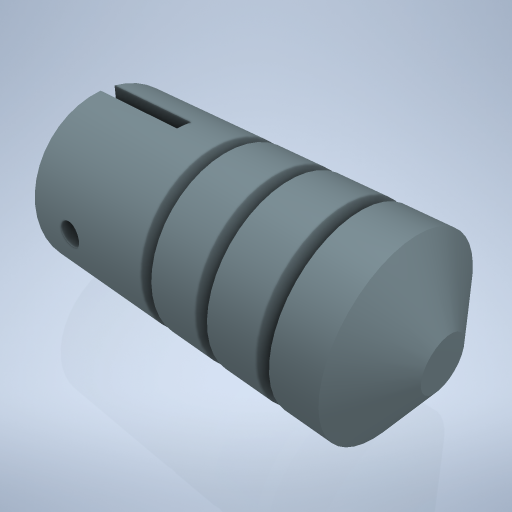
# Autodesk Inventor part: arbeitskolben
Saved by Autodesk Inventor 2024.2 (Build 282272000, 272)
## iProperties
Created: 2024-04-15
Part Number: arbeitskolben
Material: Blei
Document SubType Name: Modeling
Designer: Fabri
Density: 11.34 g/cm^3
Appearance: Blei
Author: Fabri
Autodesk Inventor part; units mm, degrees
ref_plane "YZ Plane" through (0, 0, 0) normal (1, 0, 0) x (0, 1, 0)
ref_plane "XY Plane" through (0, 0, 0) normal (0, 0, 1) x (1, 0, 0)
sketch "Skizze4" plane through (0, 0, 0) normal (0, 0, 1) x (1, 0, 0)
  line L0 (0, 0) -> (0, 7)
  line L1 (0, 7) -> (11.5, 7)
  line L2 (11.5, 7) -> (12, 6.134)
  line L3 (12, 6.134) -> (12.5, 7)
  line L4 (12.5, 7) -> (16.5, 7)
  line L5 (16.5, 7) -> (17, 6.134)
  line L6 (17, 6.134) -> (17.5, 7)
  line L7 (17.5, 7) -> (21.5, 7)
  line L8 (21.5, 7) -> (22, 6.134)
  line L9 (22, 6.134) -> (22.5, 7)
  line L10 (22.5, 7) -> (26.1132, 7)
  line L11 (26.1132, 7) -> (29, 2)
  line L12 (29, 2) -> (29, 0)
  line L13 (29, 0) -> (0, 0)
  line L14 (12, 6.134) -> (12, 7.9514) construction
  line L15 (17, 6.134) -> (17, 8.1262) construction
  line L16 (22, 6.134) -> (22, 7.8166) construction
  point P0 (29, 1)
  dimension "d7" = 1
  dimension "d8" = 60
  dimension "d9" = 4
  dimension "d10" = 14
  dimension "d11" = 7
  dimension "d12" = 29
  dimension "d13" = 12
  dimension "d14" = 17
  dimension "d15" = 30
  dimension "d16" = 1
  constraints: 34 end point, 6 point on line, 5 parallel, 4 vertical, 3 symmetric about line, 2 perpendicular, 1 horizontal alignment, 1 midpoint
  measures "d7" distance of L3.end L1.end
  measures "d8" angle of L3 L2
  measures "d9" diameter of L11.end L13
  measures "d10" diameter of L10.end L13
  measures "d11" distance from line of L12 L8.end
  measures "d12" distance between parallel lines of L12 L0
  measures "d13" horizontal distance of point (29, 1) L5.end
  measures "d14" distance from line of L12 L2.end
  measures "d15" angle of L11 L12
  measures "d16" distance of L9.end L7.end
revolve "Umdrehung1" add sketch "Skizze4" angle 360 about axis through (29, 0, 0) along (-1, 0, 0)
sketch "Skizze5" plane through (0, 0, 0) normal (-1, 0, 0) x (0, 0, 1)
  circle A0 centre (0, 0) radius 7 projected
  line L0 (-7, 0.6) -> (7, 0.6)
  line L1 (7, 0.6) -> (7, -0.6)
  line L2 (7, -0.6) -> (-7, -0.6)
  line L3 (-7, -0.6) -> (-7, 0.6)
  circle A1 centre (0, 0) radius 7 projected
  line L4 (-7, 0) -> (7.2864, 0) construction
  dimension "d18" = 1.2
  constraints: 10 end point, 2 parallel, 2 perpendicular, 2 vertical, 1 horizontal, 1 horizontal alignment, 1 midpoint, 2 other
  measures "d18" distance between parallel lines of L2 L0
extrude "Extrusion1" cut sketch "Skizze5" against normal blind 8 contours A0 L2 L0 | L1 L2 A0 | A0 L0 L1 | A0 L3 L0 | L2 L3 A0
ref_plane "Arbeitsebene1" through (0, 0, 0) normal (0, 1, 0) x (-1, 0, 0)
sketch "Skizze6" plane through (0, 0, 0) normal (0, 1, 0) x (-1, 0, 0)
  point P0 (0, 0)
  point P1 (-4, 0)
  dimension "d22" = 4
  constraints: 1 horizontal alignment
  measures "d22" distance of point (-4, 0) point (0, 0)
hole "Bohrung1" at (4, 0, 0) direction (0, -1, 0) diameter 2 end through all both
